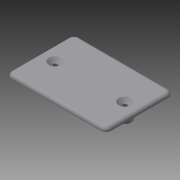
# Autodesk Inventor part: top
Saved by Autodesk Inventor 2014 (Build 180170000, 170)
## iProperties
Created: 2018-03-26
Part Number: top
Material: Generic
Document SubType Name: Modeling
Designer: HP820
Density: 1 g/cm^3
Appearance: Default
Author: HP820
Autodesk Inventor part; units mm, degrees
ref_plane "YZ Plane" through (0, 0, 0) normal (1, 0, 0) x (0, 1, 0)
ref_plane "XZ Plane" through (0, 0, 0) normal (0, 1, 0) x (-1, 0, 0)
ref_plane "XY Plane" through (0, 0, 0) normal (0, 0, 1) x (1, 0, 0)
sketch "Sketch1" plane through (0, 0, 0) normal (0, 0, 1) x (1, 0, 0)
  line L0 (24.7, 16.2) -> (24.7, -16.2) projected
  line L1 (24.7, -16.2) -> (-24.7, -16.2) projected
  line L2 (-24.7, -16.2) -> (-24.7, 16.2) projected
  line L3 (-24.7, 16.2) -> (24.7, 16.2) projected
  arc A0 (26.5, 15) -> (23.5, 18) centre (23.5, 15) ccw projected
  line L4 (23.5, 18) -> (-23.5, 18) projected
  arc A1 (-23.5, 18) -> (-26.5, 15) centre (-23.5, 15) ccw projected
  line L5 (-26.5, 15) -> (-26.5, -15) projected
  arc A2 (-26.5, -15) -> (-23.5, -18) centre (-23.5, -15) ccw projected
  line L6 (-23.5, -18) -> (23.5, -18) projected
  arc A3 (23.5, -18) -> (26.5, -15) centre (23.5, -15) ccw projected
  line L7 (26.5, -15) -> (26.5, 15) projected
  point P0 (0, 0)
extrude "Extrusion1" add sketch "Sketch1" along normal blind 1.8 contours L0 L1 L2 L3 | L7 A3 L6 A2 L5 A1 L4 A0
sketch "Sketch2" plane through (0, 0, 1.8) normal (0, 0, 1) x (1, 0, 0)
  circle A0 centre (-18.5, 0) radius 1.3 projected
  circle A1 centre (18.5, 0) radius 1.3 projected
  point P0 (0, 0)
extrude "Extrusion2" cut sketch "Sketch2" against normal blind 1.8
sketch "Sketch3" plane through (0, 0, 0) normal (0, 0, -1) x (-1, 0, 0)
  circle A0 centre (18.5, 0) radius 1.3 projected
  circle A1 centre (-18.5, 0) radius 1.3 projected
  circle A2 centre (-18.5, 0) radius 3.5
  circle A3 centre (18.5, 0) radius 3.5
  point P0 (0, 0)
  dimension "d4" = 7
  dimension "d5" = 7
  constraints: 2 centre point, 2 coincident
  measures "d4" diameter of A2
  measures "d5" diameter of A3
extrude "Extrusion3" add sketch "Sketch3" along normal blind 6.05
fillet "Fillet1" radius 1.8 8 edges at (-25.6213, 17.1213, 1.8) (-26.5, 0, 1.8) (-25.6213, -17.1213, 1.8) (0, -18, 1.8) (25.6213, -17.1213, 1.8) (26.5, 0, 1.8) (25.6213, 17.1213, 1.8) (0, 18, 1.8)
chamfer "Chamfer1" distance 2 angle 45 2 edges at (17.2, 0, 1.8) (-19.8, 0, 1.8)
body "Solid1"
